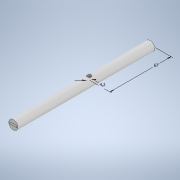
# Autodesk Inventor part: Stange1Mitte
Saved by Autodesk Inventor 2020.3 (Build 243373000, 373)
## iProperties
Created: 2020-11-29
Part Number: Stange1Mitte
Material: Generisch
Document SubType Name: Modeling
Designer: Stefan
Density: 1 g/cm^3
Appearance: Vorgabe
Author: Stefan
Autodesk Inventor part; units mm, degrees
ref_plane "YZ Plane" through (0, 0, 0) normal (1, 0, 0) x (0, 1, 0)
ref_plane "XZ Plane" through (0, 0, 0) normal (0, 1, 0) x (-1, 0, 0)
ref_plane "XY Plane" through (0, 0, 0) normal (0, 0, 1) x (1, 0, 0)
sketch "Skizze1" plane through (0, 0, 0) normal (0, 0, 1) x (1, 0, 0)
  circle A0 centre (0, 0) radius 5
  dimension "d0" = 10
  constraints: 1 centre point, 1 coincident
  measures "d0" diameter of A0
extrude "Extrusion1" add sketch "Skizze1" along normal blind 150
sketch "Skizze2" plane through (0, 0, 150) normal (0, 0, 1) x (1, 0, 0)
  line L0 (3.9734, -0.9619) -> (-4.0266, -0.9619)
  line L1 (-4.0266, -0.9619) -> (-4.0266, 1.0381)
  line L2 (-4.0266, 1.0381) -> (3.9734, 1.0381)
  line L3 (3.9734, 1.0381) -> (3.9734, -0.9619)
  point P0 (0, 0)
  dimension "d3" = 8
  dimension "d4" = 2
  constraints: 8 end point, 2 parallel, 1 horizontal, 1 perpendicular
  measures "d3" distance of L1.end L2.end
  measures "d4" distance of L0.end L1.end
extrude "Extrusion2" add sketch "Skizze2" against normal up to surface (150 mm away) separate body
sketch "Skizze3" plane through (-4.0266, 1.0381, 150) normal (0, 1, 0) x (1, 0, 0)
  circle A0 centre (4.0266, 83) radius 2.1
  line L0 (-0.9734, 150) -> (9.0266, 150) projected
  point P0 (4.0266, 150)
  dimension "d7" = 4.2
  dimension "d8" = 67
  constraints: 1 centre point
  measures "d7" diameter of A0
  measures "d8" distance from line of L0 A0.centre
extrude "Extrusion3" add sketch "Skizze3" along normal mid plane 20 separate body
combine bodies "Kombinieren1" operation type subtract main body 1 bodies to subtract 3
extrude "Extrusion4" cut sketch "Skizze3" along normal mid plane 20 bodies 2
